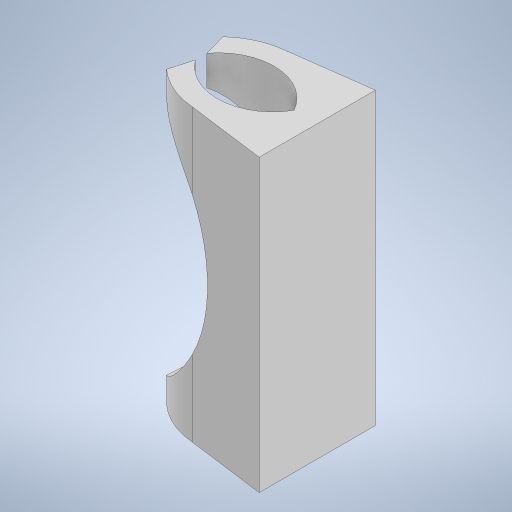
# Autodesk Inventor part: round dichroic holder
Saved by Autodesk Inventor 2024 (Build 280153000, 153)
## iProperties
Created: 2024-11-13
Part Number: round dichroic holder
Material: Generic
Document SubType Name: Modeling
Designer: Williamow
Density: 1 g/cm^3
Appearance: Default
Author: Williamow
Autodesk Inventor part; units mm, degrees
ref_plane "YZ Plane" through (0, 0, 0) normal (1, 0, 0) x (0, 1, 0)
ref_plane "XZ Plane" through (0, 0, 0) normal (0, 1, 0) x (-1, 0, 0)
ref_plane "XY Plane" through (0, 0, 0) normal (0, 0, 1) x (1, 0, 0)
sketch "Sketch1" plane through (0, 0, 0) normal (0, 1, 0) x (-1, 0, 0)
  line L0 (0, 0) -> (0.8, 0)
  arc A0 (4, 0.2) -> (0.8, 0) centre (2.4646, -0.934) ccw
  line L1 (4, 0.2) -> (4.2175, 0.9699)
  arc A1 (4.2175, 0.9699) -> (2.6673, 1.646) centre (2.4646, -0.934) ccw
  line L2 (2.6673, 1.646) -> (0, 2)
  line L3 (0, 2) -> (0, 0)
  arc A2 (0.8, 0) -> (4, -0.2) centre (2.4646, 0.934) ccw
  line L4 (4, -0.2) -> (4.2175, -0.9699)
  arc A3 (2.6673, -1.646) -> (4.2175, -0.9699) centre (2.4646, 0.934) ccw
  line L5 (2.6673, -1.646) -> (0, -2)
  line L6 (0, -2) -> (0, 0)
  dimension "d0" = 0.2
  dimension "d1" = 4
  dimension "d2" = 0.8
  dimension "d3" = 2
  dimension "d4" = 0.8
  constraints: 14 end point, 8 point on circle, 6 symmetric about line, 4 centre point, 2 coincident, 1 horizontal, 1 vertical, 2 other
  measures "d0" vertical distance of L0.end L1.start
  measures "d1" horizontal distance of L0.start L1.start
  measures "d2" distance of L1.start L1.end
  measures "d3" distance of L2.end L0.start
  measures "d4" distance of L0.start L0.end
sketch "Sketch2" plane through (0, 0, 0) normal (0, 0, 1) x (1, 0, 0)
  circle A0 centre (-7.05, 0) radius 5
  point P0 (0, 0)
  point P1 (-0.8, 0)
  dimension "d5" = 10
  dimension "d6" = 6.25
  constraints: 1 centre point, 1 horizontal alignment
  measures "d5" diameter of A0
  measures "d6" distance of point (-0.8, 0) A0.centre
extrude "Extrusion1" add sketch "Sketch1" along normal mid plane 10
extrude "Extrusion2" cut sketch "Sketch2" along normal mid plane 10
body "Solid1"
